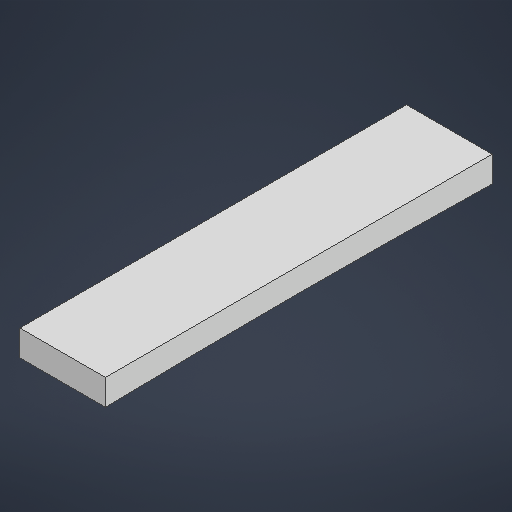
# Autodesk Inventor part: CessAssemBatteryipt
Saved by Autodesk Inventor 2027 (Build 310192060, 192F)
## iProperties
Created: 2026-07-16
Part Number: CessAssemBatteryipt
Material: Generic
Document SubType Name: Modeling
Designer: sunsh
Density: 1 g/cm^3
Appearance: Default
Author: sunsh
Autodesk Inventor part; units mm, degrees
ref_plane "YZ Plane" through (0, 0, 0) normal (1, 0, 0) x (0, 1, 0)
ref_plane "XZ Plane" through (0, 0, 0) normal (0, 1, 0) x (-1, 0, 0)
ref_plane "XY Plane" through (0, 0, 0) normal (0, 0, 1) x (1, 0, 0)
sketch "Sketch1" plane through (0, 0, 0) normal (0, 1, 0) x (-1, 0, 0)
  line L0 (387.5, 1749.9965) -> (-387.5, 1749.9965)
  line L1 (-387.5, 1749.9965) -> (-387.5, -1749.9965)
  line L2 (-387.5, -1749.9965) -> (387.5, -1749.9965)
  line L3 (387.5, -1749.9965) -> (387.5, 1749.9965)
  point P0 (0, 0)
  dimension "d0" = 3499.993
  dimension "d2" = 775
  constraints: 8 end point, 2 parallel, 1 horizontal, 1 perpendicular
  measures "d0" distance of L2.end L0.start
  measures "d2" distance of L1.end L2.end
extrude "Extrusion1" add sketch "Sketch1" along normal blind 254
sketch "Sketch2" plane through (0, 0, 0) normal (1, 0, 0) x (0, 1, 0)
  arc A0 (20.2692, -1749.9965) -> (20.2692, 1749.9965) centre (-81203.365, 0) ccw
  line L0 (0, 1749.9965) -> (0, -1749.9965) projected
  line L1 (254, -1749.9965) -> (254, 1749.9965) projected
  line L2 (20.2692, 1749.9965) -> (20.2692, -1749.9965)
  line L3 (20.2692, 1749.9965) -> (0, 1749.9965)
  point P0 (0, 0)
  dimension "d5" = 81242.4842
  dimension "d6" = 3499.993
  dimension "d7" = 233.7308
  dimension "d10" = 233.7308
  constraints: 4 end point, 2 point on circle, 1 centre point, 1 perpendicular
  measures "d5" radius of A0
  measures "d6" distance of L2.end L2.start
  measures "d7" distance from line of L1 L2.end
  measures "d10" distance from line of L1 L2.start
extrude "Extrusion2" cut sketch "Sketch2" along normal blind 1057.275 and the other way blind 885.825
sketch "Sketch4" plane through (-387.5, 0, -1749.9965) normal (-1, 0, 0) x (0, 0, 1)
  line L0 (0, 0) -> (3499.993, 0) projected
  line L1 (3499.993, 20.2692) -> (0, 20.2692) projected
  line L2 (3499.993, 0) -> (3499.993, 20.2692) projected
  line L3 (0, 0) -> (0, 20.2692) projected
  point P0 (1749.9965, 0)
extrude "Extrusion3" cut sketch "Sketch4" against normal through all
shell "Shell1" thickness 25.4 removed faces 1 at (129.1667, 22.9583, -1620.385)
body "Solid1"
